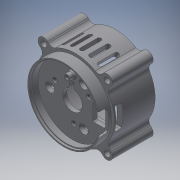
# Autodesk Inventor part: motor_mount_with_motor_driver
Saved by Autodesk Inventor 2019.4 (Build 234330000, 330)
## iProperties
Created: 2019-06-20
Part Number: motor_mount_with_motor_driver
Material: Generic
Document SubType Name: Modeling
Designer: cdi
Density: 1 g/cm^3
Appearance: Default
Author: cdi
Autodesk Inventor part; units mm, degrees
ref_plane "YZ Plane" through (0, 0, 0) normal (1, 0, 0) x (0, 1, 0)
ref_plane "XZ Plane" through (0, 0, 0) normal (0, 1, 0) x (-1, 0, 0)
sketch "Sketch1" plane through (0, 0, 0) normal (0, 0, 1) x (1, 0, 0)
  circle A0 centre (0, 0) radius 28
  dimension "d0" = 56
  constraints: 1 centre point, 1 coincident
  measures "d0" diameter of A0
extrude "Extrusion1" add sketch "Sketch1" along normal blind 3
sketch "Sketch2" plane through (0, 0, 3) normal (0, 0, 1) x (1, 0, 0)
  circle A0 centre (0, 0) radius 7
  dimension "d3" = 14
  constraints: 1 centre point, 1 coincident
  measures "d3" diameter of A0
extrude "Extrusion2" cut sketch "Sketch2" against normal through all
sketch "Sketch3" plane through (0, 0, 0) normal (0, 0, -1) x (-1, 0, 0)
  circle A0 centre (0, 0) radius 24
  circle A1 centre (0, 0) radius 28 projected
  dimension "d6" = 48
  dimension "d7" = 4
  constraints: 1 centre point, 1 coincident
  measures "d6" diameter of A0
  measures "d7" radial gap between concentric circles of A1 A0
extrude "Extrusion3" add sketch "Sketch3" along normal blind 5
sketch "Sketch4" plane through (0, 0, 3) normal (0, 0, 1) x (1, 0, 0)
  circle A0 centre (0, 0) radius 10.25
  circle A1 centre (0, 0) radius 12.475
  dimension "d11" = 20.5
  dimension "d121" = 24.95
  constraints: 2 centre point, 2 coincident
  measures "d11" diameter of A0
  measures "d121" diameter of A1
extrude "Extrusion4" add sketch "Sketch4" along normal blind 5
sketch "Sketch5" plane through (0, 0, 3) normal (0, 0, 1) x (1, 0, 0)
  circle A0 centre (0, 0) radius 10.25
  circle A1 centre (0, 0) radius 9
  dimension "d15" = 18
  constraints: 2 centre point, 2 coincident
  measures "d15" diameter of A1
extrude "Extrusion5" add sketch "Sketch5" along normal blind 3.5
sketch "Sketch6" plane through (0, 0, 3) normal (0, 0, 1) x (1, 0, 0)
  circle A0 centre (0, 0) radius 8.5
  circle A1 centre (0, 8.5) radius 1.5
  circle A2 centre (0, -8.5) radius 1.5
  dimension "d18" = 17
  dimension "d19" = 3
  dimension "d20" = 3
  constraints: 3 centre point, 2 point on circle, 1 coincident
  measures "d18" diameter of A0
  measures "d19" diameter of A1
  measures "d20" diameter of A2
extrude "Extrusion6" add sketch "Sketch6" along normal blind 3.5 contours A1 A0 | A0 A1 | A2 A0 | A0 A2
sketch "Sketch7" plane through (0, 0, 6.5) normal (0, 0, 1) x (1, 0, 0)
  arc A0 (1.4505, -8.8824) -> (-1.4505, -8.8824) centre (0, -8.5) ccw projected
  arc A1 (-1.4505, 8.8824) -> (1.4505, 8.8824) centre (0, 8.5) ccw projected
  circle A2 centre (0, -8.5) radius 0.75
  circle A3 centre (0, 8.5) radius 0.75
  point P0 (0, 0)
  dimension "d23" = 1.5
  dimension "d24" = 1.5
  constraints: 2 centre point, 2 coincident
  measures "d23" diameter of A2
  measures "d24" diameter of A3
hole "Hole1" [suppressed]
sketch "Sketch8" plane through (0, 0, 3) normal (0, 0, 1) x (1, 0, 0)
  circle A0 centre (0, 0) radius 16
  circle A1 centre (-16, 0) radius 1.5
  dimension "d32" = 32
  dimension "d33" = 3
  constraints: 1 centre point, 1 coincident, 1 horizontal alignment, 2 other
  measures "d33" diameter of A1
extrude "Extrusion7" cut sketch "Sketch8" against normal through all contours A1 A0 | A0 A1 picked at (-15.4948, 0) picked at (-16.4909, 0.0621)
pattern_circular "Circular Pattern1" count 3 over 360 about axis through (0, 0, 3) along (0, 0, 1) of "Extrusion7"
sketch "Sketch9" plane through (0, 0, 0) normal (0, 0, -1) x (-1, 0, 0)
  line L0 (0, -8) -> (-37.4126, -8)
  line L1 (-37.4126, -8) -> (-37.4126, 8)
  line L2 (-37.4126, 8) -> (0, 8)
  line L3 (0, 8) -> (0, -8)
  point P0 (0, 0)
  dimension "d39" = 16
  dimension "d40" = 8
  constraints: 8 end point, 2 parallel, 1 horizontal, 1 perpendicular
  measures "d39" distance of L2.end L0.start
  measures "d40" distance from line of point (0, 0) L2
extrude "Extrusion8" cut sketch "Sketch9" along normal blind 5
sketch "Sketch10" plane through (0, 0, -5) normal (0, 0, -1) x (-1, 0, 0)
  circle A0 centre (0, 0) radius 28
  circle A1 centre (0, 0) radius 24
  arc A2 (-26.8328, -8) -> (-26.8328, 8) centre (0, 0) ccw projected
  dimension "d46" = 0
  dimension "d80" = 48
  constraints: 2 centre point, 2 coincident
  measures "d46" radial gap between concentric circles of A2 A0
  measures "d80" diameter of A1
extrude "Extrusion9" add sketch "Sketch10" along normal blind 18
fillet "Fillet1" radius 2 1 edges at (-28, 0, 3)
sketch "Sketch12" plane through (0, 0, -23) normal (0, 0, -1) x (-1, 0, 0)
  circle A0 centre (0, 0) radius 26.04
  dimension "d56" = 52.08
  constraints: 1 centre point, 1 coincident
  measures "d56" diameter of A0
extrude "Extrusion10" cut sketch "Sketch12" against normal blind 3
sketch "Sketch13" plane through (0, 0, -23) normal (0, 0, -1) x (-1, 0, 0)
  circle A0 centre (0, 0) radius 26.04 projected
  circle A1 centre (0, 0) radius 28 projected
extrude "Extrusion11" add sketch "Sketch13" along normal blind 5
sketch "Sketch14" plane through (0, 0, -28) normal (0, 0, -1) x (-1, 0, 0)
  circle A0 centre (0, 0) radius 28 projected
  arc A1 (-26.8328, 8) -> (-26.8328, -8) centre (0, 0) ccw projected
  arc A2 (-26.8328, 8) -> (-26.8328, -8) centre (0, 0) ccw projected
  circle A3 centre (0, 0) radius 28 projected
  circle A4 centre (32, 0) radius 1.5
  circle A5 centre (22.6274, 22.6274) radius 1.5
  circle A6 centre (0, 32) radius 1.5
  circle A7 centre (-22.6274, 22.6274) radius 1.5
  circle A8 centre (-32, 0) radius 1.5
  circle A9 centre (-22.6274, -22.6274) radius 1.5
  circle A10 centre (0, -32) radius 1.5
  circle A11 centre (22.6274, -22.6274) radius 1.5
  arc A12 (19.799, -25.4558) -> (25.4558, -19.799) centre (22.6274, -22.6274) ccw
  line L0 (22.6274, -22.6274) -> (0, 0)
  line L1 (25.4558, -19.799) -> (22.4243, -16.7675)
  line L2 (19.799, -25.4558) -> (16.7675, -22.4243)
  arc A13 (16.7675, -22.4243) -> (22.4243, -16.7675) centre (0, 0) ccw
  dimension "d61" = 3
  dimension "d62" = 32
  dimension "d65" = 360
  constraints: 10 centre point, 6 end point, 6 point on circle, 3 tangent, 2 parallel, 1 coincident, 17 other
  measures "d61" diameter of A4
  measures "d62" distance of point (0, 0) A4.centre
extrude "Extrusion12" add sketch "Sketch14" against normal blind 29 contours L1 A12 L2 A0
fillet "Fillet2" radius 4 2 edges at (-22.4243, -16.7675, -13.5) (-16.7675, -22.4243, -13.5)
pattern_circular "Circular Pattern2" count 4 over 360 about axis through (0, 0, 0) along (0, 0, 1) of "Extrusion12", "Fillet2"
sketch "Sketch15" plane through (0, 0, -28) normal (0, 0, -1) x (-1, 0, 0)
  circle A0 centre (22.6274, 22.6274) radius 1.5 projected
  circle A1 centre (-22.6274, 22.6274) radius 1.5 projected
  circle A2 centre (-22.6274, -22.6274) radius 1.5 projected
  circle A3 centre (22.6274, -22.6274) radius 1.5 projected
  circle A4 centre (0, 0) radius 26.04 projected
  arc A5 (24.12, -14.2205) -> (24.12, 14.2205) centre (0, 0) ccw projected
  arc A6 (24.7373, 19.0805) -> (24.12, 14.2205) centre (27.5658, 16.252) ccw projected
  arc A7 (25.4558, 19.799) -> (19.799, 25.4558) centre (22.6274, 22.6274) ccw projected
  arc A8 (14.2205, 24.12) -> (19.0805, 24.7373) centre (16.252, 27.5658) ccw projected
  arc A9 (14.2205, 24.12) -> (-14.2205, 24.12) centre (0, 0) ccw projected
  arc A10 (-19.0805, 24.7373) -> (-14.2205, 24.12) centre (-16.252, 27.5658) ccw projected
  arc A11 (-19.799, 25.4558) -> (-25.4558, 19.799) centre (-22.6274, 22.6274) ccw projected
  arc A12 (-24.12, 14.2205) -> (-24.7373, 19.0805) centre (-27.5658, 16.252) ccw projected
  arc A13 (-24.12, 14.2205) -> (-24.12, -14.2205) centre (0, 0) ccw projected
  arc A14 (-24.7373, -19.0805) -> (-24.12, -14.2205) centre (-27.5658, -16.252) ccw projected
  arc A15 (-25.4558, -19.799) -> (-19.799, -25.4558) centre (-22.6274, -22.6274) ccw projected
  arc A16 (-14.2205, -24.12) -> (-19.0805, -24.7373) centre (-16.252, -27.5658) ccw projected
  arc A17 (-14.2205, -24.12) -> (14.2205, -24.12) centre (0, 0) ccw projected
  arc A18 (19.0805, -24.7373) -> (14.2205, -24.12) centre (16.252, -27.5658) ccw projected
  arc A19 (19.799, -25.4558) -> (25.4558, -19.799) centre (22.6274, -22.6274) ccw projected
  arc A20 (24.12, -14.2205) -> (24.7373, -19.0805) centre (27.5658, -16.252) ccw projected
  line L0 (24.7373, 19.0805) -> (25.4558, 19.799) projected
  line L1 (19.799, 25.4558) -> (19.0805, 24.7373) projected
  line L2 (-19.0805, 24.7373) -> (-19.799, 25.4558) projected
  line L3 (-25.4558, 19.799) -> (-24.7373, 19.0805) projected
  line L4 (-24.7373, -19.0805) -> (-25.4558, -19.799) projected
  line L5 (-19.799, -25.4558) -> (-19.0805, -24.7373) projected
  line L6 (19.0805, -24.7373) -> (19.799, -25.4558) projected
  line L7 (25.4558, -19.799) -> (24.7373, -19.0805) projected
hole "Hole2" at (22.6274, 22.6274, -28) at (-22.6274, 22.6274, -28) at (-22.6274, -22.6274, -28) at (22.6274, -22.6274, -28) direction (0, 0, 1) diameter 3.88 depth 10 tip angle 118 countersink diameter 4.34 countersink angle 7
fillet "Fillet3" radius 2 1 edges at (-24, 0, 0)
sketch "Sketch17" plane through (0, 0, 3) normal (0, 0, 1) x (1, 0, 0)
  line L0 (0, 0) -> (46.0168, 0)
  arc A0 (21, -1.5) -> (21, 1.5) centre (21, 0) ccw
  arc A1 (15, 1.5) -> (15, -1.5) centre (15, 0) ccw
  line L1 (21, 1.5) -> (15, 1.5)
  line L2 (21, -1.5) -> (15, -1.5)
  dimension "d82" = 3
  dimension "d83" = 3
  dimension "d84" = 6
  dimension "d85" = 15
  constraints: 6 end point, 4 point on circle, 2 centre point, 2 point on line, 2 tangent, 1 horizontal
  measures "d82" diameter of A0
  measures "d83" diameter of A1
  measures "d84" distance of A0.centre A1.centre
  measures "d85" distance of L0.start A1.centre
extrude "Extrusion13" [suppressed]
pattern_circular "Circular Pattern3" [suppressed]
mirror "Mirror1" [suppressed]
pattern_circular "Circular Pattern4" [suppressed]
ref_plane "Work Plane1" through (0, 0, -13.5) normal (0, 0, -1) x (-1, 0, 0)
mirror "Mirror2" about plane through (0, 0, -13.5) normal (0, 0, -1) of "Hole2"
sketch "Sketch18" plane through (0, 0, 1) normal (0, 0, 1) x (0.7071068, -0.7071068, 0)
  circle A0 centre (32, 0) radius 1.5 projected
  circle A1 centre (32, 0) radius 1.94
  point P0 (0, 0)
  dimension "d94" = 3.88
  constraints: 1 centre point, 1 coincident
  measures "d94" diameter of A1
extrude "Extrusion14" cut sketch "Sketch18" against normal through all contours A0 | A1
pattern_circular "Circular Pattern5" count 4 over 360 about axis through (0, 0, 0) along (0, 0, 1) of "Extrusion14"
sketch "Sketch19" plane through (0, 0, 0) normal (1, 0, 0) x (0, 1, 0)
  line L0 (0, 0) -> (0, -16)
  arc A0 (-1.5, -16) -> (1.5, -16) centre (0, -16) ccw
  arc A1 (1.5, -4) -> (-1.5, -4) centre (0, -4) ccw
  line L1 (-1.5, -4) -> (-1.5, -16)
  line L2 (1.5, -16) -> (1.5, -4)
  dimension "d100" = 16
  dimension "d101" = 3
  dimension "d102" = 3
  dimension "d103" = 12
  dimension "d176" = 4
  constraints: 6 end point, 4 point on circle, 2 centre point, 2 tangent, 1 coincident, 1 point on line, 1 vertical
  measures "d100" distance of L0.start L0.end
  measures "d101" diameter of A0
  measures "d102" diameter of A1
  measures "d103" distance of A0.centre A1.centre
  measures "d176" distance of A1.centre L0.start
extrude "Extrusion15" cut sketch "Sketch19" against normal blind 40
pattern_circular "Circular Pattern6" count 3 over 27 about axis through (0, 0, 0) along (0, 0, 1) of "Extrusion15"
mirror "Mirror3" about plane through (0, 0, 0) normal (0, 1, 0) of "Extrusion15", "Circular Pattern6"
pattern_circular "Circular Pattern7" count 2 over 90 about axis through (0, 0, 0) along (0, 0, 1) of "Extrusion15", "Circular Pattern6", "Mirror3"
mirror "Mirror4" about plane through (0, 0, 0) normal (0, 1, 0) of "Extrusion15", "Circular Pattern6", "Mirror3", "Circular Pattern7"
fillet "Fillet5" radius 1 4 edges at (23.6634, 8, 0) (23.6634, -8, 0) (24.7301, -8, -5) (24.7301, 8, -5)
sketch "Sketch20" plane through (0, 0, 3) normal (0, 0, 1) x (1, 0, 0)
  circle A0 centre (-16, 0) radius 1.5 projected
  circle A1 centre (8, 13.8564) radius 1.5 projected
  circle A2 centre (8, -13.8564) radius 1.5 projected
  point P0 (0, 0)
hole "Hole3" at (8, 13.8564, 3) at (-16, 0, 3) at (8, -13.8564, 3) direction (0, 0, -1) diameter 3.1 depth 10 countersink diameter 6.5 countersink angle 90
sketch "스케치21" plane through (0, 0, 8) normal (0, 0, 1) x (1, 0, 0)
  circle A0 centre (0, 0) radius 12.475
  constraints: 1 centre point, 1 coincident
extrude "돌출16" cut sketch "스케치21" against normal up to surface (5 mm away)
sketch "스케치22" plane through (0, 0, 3) normal (0, 0, 1) x (1, 0, 0)
  circle A0 centre (0, 16) radius 2
  line L0 (0, 0) -> (0, 3.2224)
  line L1 (0, 16) -> (0, 0)
  dimension "d124" = 4
  dimension "d125" = 16
  dimension "d138" = 0
  constraints: 4 end point, 1 centre point, 1 vertical
  measures "d124" diameter of A0
  measures "d125" distance of L0.start L1.start
  measures "d138" distance between parallel lines of L1 L0
extrude "돌출17" add sketch "스케치22" along normal blind 4
sketch "스케치23" plane through (0, 0, 3) normal (0, 0, 1) x (1, 0, 0)
  circle A0 centre (0, 0) radius 24.5
  circle A1 centre (0, 0) radius 26
  dimension "d131" = 49
  dimension "d132" = 52
  constraints: 2 centre point, 2 coincident
  measures "d131" diameter of A0
  measures "d132" diameter of A1
extrude "돌출18" add sketch "스케치23" along normal blind 6
sketch "스케치24" plane through (0, 0, 9) normal (0, 0, 1) x (1, 0, 0)
  circle A0 centre (0, 0) radius 25.15
  dimension "d135" = 50.3
  constraints: 1 centre point, 1 coincident
  measures "d135" diameter of A0
extrude "돌출19" cut sketch "스케치24" against normal blind 1.6
fillet "모깎기6" radius 1 1 edges at (-2, 16, 3)
sketch "스케치26" plane through (0, 0, 3) normal (0, 0, 1) x (1, 0, 0)
  line L0 (14.5, -6) -> (23.5, -6)
  line L1 (23.5, -6) -> (23.5, 6)
  line L2 (23.5, 6) -> (14.5, 6)
  line L3 (14.5, 6) -> (14.5, -6)
  line L4 (14.5, -6) -> (23.5, 6) construction
  line L5 (23.5, -6) -> (14.5, 6) construction
  point P0 (0, 0)
  point P1 (19, 0)
  dimension "d150" = 9
  dimension "d151" = 12
  dimension "d152" = 19
  constraints: 12 end point, 2 midpoint, 2 parallel, 1 horizontal, 1 perpendicular
  measures "d150" distance of L2.end L1.end
  measures "d151" distance of L1.end L0.end
  measures "d152" distance of point (0, 0) point (19, 0)
extrude "돌출20" cut sketch "스케치26" against normal up to surface (3 mm away)
fillet "모깎기7" radius 1 4 edges at (23.5, -6, 1.5) (14.5, -6, 1.5) (14.5, 6, 1.5) (23.5, 6, 1.5)
sketch "스케치28" plane through (0, 0, 3) normal (0, 0, 1) x (1, 0, 0)
  circle A0 centre (0, 0) radius 7 projected
  line L0 (-2.1, 6.6776) -> (1.4, 6.6776)
  line L1 (1.4, 6.6776) -> (1.4, 11.8776)
  line L2 (1.4, 11.8776) -> (-2.1, 11.8776)
  line L3 (-2.1, 11.8776) -> (-2.1, 6.6776)
  dimension "d163" = 2.1
  dimension "d164" = 3.5
  dimension "d165" = 5.2
  constraints: 8 end point, 2 parallel, 1 horizontal, 1 perpendicular, 2 other
  measures "d163" distance from line of point (0, 0) L3
  measures "d164" distance of L1.end L2.end
  measures "d165" distance of L2.end L0.start
extrude "돌출21" cut sketch "스케치28" against normal blind 10 contours L3 L2 L1 A0 | A0 L1 L0 picked at (-0.5497, 6.7635)
sketch "스케치29" plane through (0, 0, 0) normal (0, 1, 0) x (-1, 0, 0)
  line L0 (24.12, 1) -> (14.2205, 1) projected
  line L1 (14.2205, 1) -> (-14.2205, 1) projected
  line L2 (-14.2205, 1) -> (-24.12, 1) projected
  line L3 (-24.12, 1) -> (-24.12, 1) projected
  line L4 (-24.12, 1) -> (-14.2205, 1) projected
  line L5 (-14.2205, 1) -> (14.2205, 1) projected
  line L6 (14.2205, 1) -> (24.12, 1) projected
  line L7 (24.12, 1) -> (24.12, 1) projected
  line L8 (-26, 3) -> (26, 3) projected
  line L9 (-26, 3) -> (26, 3) projected
  line L10 (26, 3) -> (34.2976, 3)
  line L11 (34.2976, 3) -> (34.2976, 1)
  line L12 (34.2976, 1) -> (26, 1)
  line L13 (26, 1) -> (26, 3)
  line L14 (0, 0) -> (0, 74.1075)
  constraints: 10 end point, 2 parallel, 1 horizontal, 1 perpendicular, 1 vertical
revolve "회전1" cut sketch "스케치29" angle 360 about axis through (0, 0, 0) along (0, 0, 1)
sketch "스케치30" plane through (23.5, -5, 3) normal (-1, 0, 0) x (0, 0, 1)
  line L0 (-3, 9.9643) -> (4.4, 9.9643)
  line L1 (4.4, 9.9643) -> (4.4, 0)
  line L2 (4.4, 0) -> (-3, 0)
  line L3 (-3, 0) -> (-3, 9.9643)
  line L4 (4.4, -19.5) -> (4.4, 29.5) projected
  line L5 (4.4, 0) -> (0, 0)
  line L6 (0, 0) -> (0, 9.9643)
  line L7 (0, 9.9643) -> (4.4, 9.9643)
  line L8 (4.4, 9.9643) -> (4.4, 0)
  line L9 (0, 10) -> (0, 0) projected
  point P0 (-3, 5)
  dimension "d169" = 0
  dimension "d170" = 0
  dimension "d174" = 4.4
  constraints: 16 end point, 4 parallel, 2 horizontal, 2 perpendicular, 1 point on line
  measures "d169" distance between parallel lines of L4 L1
  measures "d170" distance between parallel lines of L9 L6
  measures "d174" distance between parallel lines of L1 L6
extrude "돌출22" cut sketch "스케치30" against normal blind 10 contours L0 L1 L2 L6
fillet "모깎기8" radius 1 4 edges at (24.7495, -5, 3) (24.7567, 4.9643, 3) (25.0884, 4.9643, 7.4) (25.0813, -5, 7.4)
fillet "모깎기9" radius 1 4 edges at (-2.1, 11.8776, 1.5) (1.4, 11.8776, 1.5) (-2.1, 6.6776, 1.5) (1.4, 6.8586, 1.5)
sketch "Sketch31" plane through (0, 16, 7) normal (0, 0, 1) x (1, 0, 0)
  circle A0 centre (0, 0) radius 2 projected
  point P0 (0, -16)
hole "Hole6" at (0, 16, 7) direction (0, 0, -1) diameter 1.713 depth 7 thread size "M2.2x0.45" class "6H" standard "ISO Metric profile"
sketch "Sketch32" plane through (0, 0, 3) normal (0, 0, 1) x (1, 0, 0)
  line L0 (23.9844, -5) -> (25.5147, -5) projected
  line L1 (25.5217, 4.9643) -> (23.9918, 4.9643) projected
  line L2 (23.5, -5) -> (30.898, -5)
  line L3 (30.898, -5) -> (30.898, 4.9643)
  line L4 (30.898, 4.9643) -> (23.5, 4.9643)
  line L5 (23.5, 4.9643) -> (23.5, -5)
  point P0 (0, 0)
  constraints: 8 end point, 2 parallel, 1 horizontal, 1 perpendicular
extrude "Extrusion23" cut sketch "Sketch32" along normal blind 10
fillet "Fillet10" radius 2 2 edges at (24.7495, -5, 3) (24.7567, 4.9643, 3)
sketch "Sketch33" plane through (0, 0, 3) normal (0, 0, 1) x (1, 0, 0)
  circle A0 centre (0, 0) radius 14
  line L0 (0, 0) -> (-12.5831, 6.1372)
  line L1 (0, 0) -> (-10.0732, 0)
  circle A1 centre (-12.5831, 6.1372) radius 1.5
  dimension "d187" = 28
  dimension "d188" = 26
  dimension "d189" = 3
  constraints: 4 end point, 2 coincident, 1 centre point, 1 horizontal, 3 other
  measures "d188" angle of L0 L1
  measures "d189" diameter of A1
hole "Hole7" at (-12.5831, 6.1372, 3) direction (0, 0, -1) diameter 2.459 depth 8.8 thread size "M3x0.5" class "6H" standard "ISO Metric profile"
pattern_circular "Circular Pattern8" count 3 over 360 about axis through (0, 0, 3) along (0, 0, -1) of "Hole7"
chamfer "Chamfer1" distance 0.5 angle 45 4 edges at (0, 16.8565, 7) (-12.5831, 7.3667, 3) (12.6713, 7.214, 3) (-0.0882, -14.5806, 3)
sketch "Sketch34" plane through (23.5, -5, 3) normal (-1, 0, 0) x (0, 0, 1)
  line L0 (0, -19.5) -> (0, 29.5) projected
  line L1 (0, -4) -> (9.8619, -4)
  line L2 (9.8619, -4) -> (9.8619, 13.9643)
  line L3 (9.8619, 13.9643) -> (0, 13.9643)
  line L4 (0, 13.9643) -> (0, -4)
  line L5 (4.4, 0) -> (2, 0) projected
  line L6 (4.4, 9.9643) -> (6, 9.9643) projected
  point P0 (-3, 5)
  point P1 (0, 7.9643)
  point P2 (0, 2)
  dimension "d204" = 4
  dimension "d205" = 4
  constraints: 8 end point, 2 parallel, 1 horizontal, 1 perpendicular, 1 point on line
  measures "d204" distance between parallel lines of L1 L5
  measures "d205" distance between parallel lines of L6 L3
extrude "Extrusion24" cut sketch "Sketch34" against normal blind 10 and the other way blind 5
fillet "Fillet12" radius 2 2 edges at (23.5898, -9, 3) (23.6034, 8.9643, 3)
body "Solid1"
